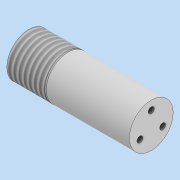
# Autodesk Inventor part: Überlast Führung
Saved by Autodesk Inventor 2021 (Build 250183000, 183)
## iProperties
Created: 2024-03-14
Part Number: Überlast Führung
Material: Generic
Document SubType Name: Modeling
Designer: Nokia
Density: 1 g/cm^3
Appearance: Default
Author: Nokia
Autodesk Inventor part; units mm, degrees
ref_plane "YZ Plane" through (0, 0, 0) normal (1, 0, 0) x (0, 1, 0)
ref_plane "XZ Plane" through (0, 0, 0) normal (0, 1, 0) x (-1, 0, 0)
ref_plane "XY Plane" through (0, 0, 0) normal (0, 0, 1) x (1, 0, 0)
sketch "Sketch1" plane through (0, 0, 0) normal (0, 0, 1) x (1, 0, 0)
  line L0 (0, 0) -> (0, 15)
  line L1 (-84, 15) -> (-84, 0)
  line L2 (-84, 0) -> (0, 0)
  arc A0 (-58, 15) -> (-57, 15) centre (-57.5, 15) ccw
  line L3 (0, 15) -> (-57, 15)
  line L4 (-58, 15) -> (-84, 15)
  dimension "d0" = 15
  dimension "d1" = 84
  constraints: 10 end point, 5 perpendicular, 2 point on circle, 1 centre point, 1 vertical
  measures "d0" distance of L0.start L0.end
  measures "d1" distance of L0.end L1.start
revolve "Revolution1" add sketch "Sketch1" angle 360 about axis through (-84, 0, 0) along (1, 0, 0)
thread "Thread1" size "M30x3.5" class "6g" standard "ANSI Metric M Profile" length 50
sketch "Sketch2" plane through (0, 0, 0) normal (1, 0, 0) x (0, 0, -1)
  circle A0 centre (0, 0) radius 15
  circle A1 centre (0, 9) radius 3.5
  circle A2 centre (-7.7942, -4.5) radius 3.5
  circle A3 centre (7.7942, -4.5) radius 3.5
  dimension "d10" = 30
  dimension "d11" = 7
  dimension "d12" = 360
  dimension "d13" = 9
  constraints: 4 centre point, 7 other
  measures "d10" diameter of A0
  measures "d11" diameter of A1
  measures "d13" distance of A1.centre point (0, 0)
hole "Hole1" at (0, 9, 0) at (0, -4.5, 7.7942) at (0, -4.5, -7.7942) direction (-1, 0, 0) diameter 4.134 depth 14.2 tip angle 118 thread size "M5x0.8" class "6H" standard "ISO Metric profile"
body "Solid1"
